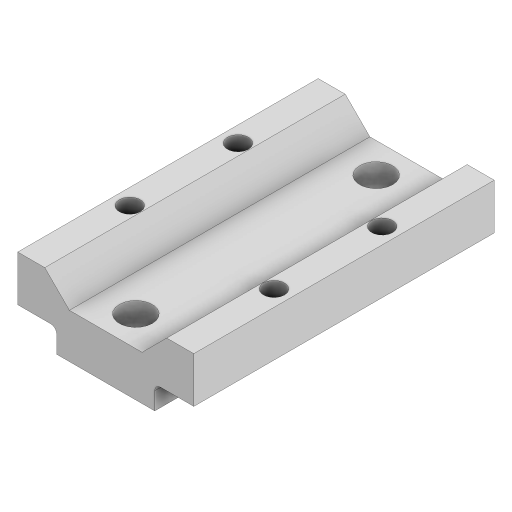
# Autodesk Inventor part: Acople_rodamiento_lineal
Saved by Autodesk Inventor 2023 (Build 270158000, 158)
## iProperties
Created: 2024-09-30
Part Number: Acople_rodamiento_lineal
Material: Generic
Document SubType Name: Modeling
Designer: diego
Density: 1 g/cm^3
Appearance: Default
Author: diego
Autodesk Inventor part; units mm, degrees
ref_plane "YZ Plane" through (0, 0, 0) normal (1, 0, 0) x (0, 1, 0)
ref_plane "XZ Plane" through (0, 0, 0) normal (0, 1, 0) x (-1, 0, 0)
ref_plane "XY Plane" through (0, 0, 0) normal (0, 0, 1) x (1, 0, 0)
sketch "Sketch1" plane through (0, 0, 0) normal (0, 0, 1) x (1, 0, 0)
  line L0 (-14.65, 5.75) -> (-10.15, 5.75)
  line L1 (-10.15, 5.75) -> (-6.05, 1.65)
  line L2 (-6.05, 1.65) -> (6.05, 1.65)
  line L3 (6.05, 1.65) -> (10.15, 5.75)
  line L4 (10.15, 5.75) -> (14.65, 5.75)
  line L5 (-14.65, 5.75) -> (-14.65, -1.85)
  line L6 (-14.65, -1.85) -> (-8.15, -1.85)
  line L7 (-8.15, -1.85) -> (-8.15, -5.75)
  line L8 (-8.15, -5.75) -> (8.15, -5.75)
  line L9 (8.15, -5.75) -> (8.15, -1.85)
  line L10 (8.15, -1.85) -> (14.65, -1.85)
  line L11 (14.65, -1.85) -> (14.65, 5.75)
  line L12 (0, -5.75) -> (0, 5.75) construction
  point P0 (0, 0)
  point P1 (0, 0)
  dimension "d0" = 12.1
  dimension "d1" = 4.5
  dimension "d2" = 135
  dimension "d3" = 7.6
  dimension "d4" = 6.5
  dimension "d6" = 4.1
  dimension "d29" = 11.5
  constraints: 26 end point, 5 perpendicular, 3 equal length, 2 horizontal, 2 midpoint, 2 point on line, 2 vertical, 1 coincident, 1 collinear, 1 horizontal alignment, 1 parallel
  measures "d0" distance of L1.end L2.end
  measures "d1" distance of L3.end L4.end
  measures "d2" angle of L2 L1
  measures "d3" distance of L10.end L4.end
  measures "d4" distance of L5.end L6.end
  measures "d6" distance between parallel lines of L0 L2
  measures "d29" distance between parallel lines of L4 L8
extrude "Extrusion1" add sketch "Sketch1" along normal mid plane 50
sketch "Sketch2" plane through (-14.65, 5.75, 25) normal (0, 1, 0) x (1, 0, 0)
  circle A0 centre (2.65, 34) radius 1.75
  line L0 (-5.86, 25) -> (35.16, 25) projected
  line L1 (14.65, 60) -> (14.65, -10) projected
  circle A1 centre (26.65, 34) radius 1.75
  circle A2 centre (2.65, 16) radius 1.75
  circle A3 centre (26.65, 16) radius 1.75
  line L2 (2.65, 16) -> (26.65, 16) construction
  line L3 (26.65, 16) -> (26.65, 34) construction
  line L4 (26.65, 34) -> (2.65, 34) construction
  line L5 (2.65, 34) -> (2.65, 16) construction
  point P0 (14.65, 25)
  point P1 (2.65, 25)
  point P2 (14.65, 34)
  dimension "d11" = 24
  dimension "d14" = 18
  dimension "d17" = 3.5
  constraints: 8 end point, 4 centre point, 2 horizontal, 2 midpoint, 2 parallel, 1 horizontal alignment, 1 perpendicular, 1 vertical, 1 vertical alignment, 6 other
  measures "d11" distance of A0.centre L3.end
  measures "d14" distance of A0.centre L2.start
  measures "d17" diameter of A0
extrude "Extrusion2" cut sketch "Sketch2" against normal through all
sketch "Sketch3" plane through (-6.05, 1.65, 25) normal (0, 1, 0) x (1, 0, 0)
  circle A0 centre (6.05, 45) radius 2.75
  circle A1 centre (6.05, 5) radius 2.75
  line L0 (6.05, 5) -> (6.05, 45) construction
  line L1 (1.7705, 10) -> (10.3295, 10)
  line L2 (10.3295, 10) -> (10.3295, 40)
  line L3 (10.3295, 40) -> (1.7705, 40)
  line L4 (1.7705, 40) -> (1.7705, 10)
  line L5 (1.7705, 10) -> (10.3295, 40) construction
  line L6 (10.3295, 10) -> (1.7705, 40) construction
  circle A2 centre (6.05, 45) radius 4.25 construction
  point P0 (6.05, 25)
  point P1 (6.05, 25)
  dimension "d21" = 5.5
  dimension "d23" = 40
  dimension "d24" = 30
  dimension "d25" = 8.5
  constraints: 14 end point, 3 centre point, 3 midpoint, 2 coincident, 2 parallel, 1 equal radius, 1 horizontal, 1 perpendicular, 1 vertical
  measures "d21" diameter of A1
  measures "d23" distance of L0.start L0.end
  measures "d24" distance of L1.end L2.end
  measures "d25" diameter of A2
extrude "Extrusion3" cut sketch "Sketch3" against normal through all contours A0 | A1
fillet "Fillet2" radius 1 2 edges at (8.15, -1.85, 0) (-8.15, -1.85, 0)
body "Solid1"
